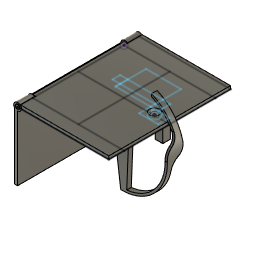
useless_machine (Autodesk Fusion 360 design; units mm, degrees)
Autodesk Fusion 360 part; units mm, degrees
sketch "Sketch1" plane through (0, 0, 0) normal (0, 0, 1) x (1, 0, 0)
  line L0 (0, 0) -> (60, 0)
  line L1 (60, 0) -> (60, -60)
  line L2 (60, -60) -> (0, -60)
  line L3 (0, -60) -> (0, 0)
  line L4 (60, -30) -> (0, -30)
  line L5 (30, 0) -> (30, -60)
  circle A0 centre (50, -30) radius 3.25
  line L6 (60, 0) -> (60, 10)
  line L7 (60, 10) -> (0, 10)
  line L8 (0, 10) -> (0, 0)
  line L9 (60, -60) -> (60, -70)
  line L10 (60, -70) -> (0, -70)
  line L11 (0, -70) -> (0, -60)
  line L12 (56.25, -26.25) -> (43.75, -26.25)
  line L13 (43.75, -26.25) -> (43.75, -33.75)
  line L14 (43.75, -33.75) -> (56.25, -33.75)
  line L15 (56.25, -33.75) -> (56.25, -26.25)
  line L16 (43.75, -26.25) -> (43.75, -23.25)
  line L17 (43.75, -23.25) -> (48.75, -23.25)
  line L18 (48.75, -23.25) -> (48.75, -18.25)
  line L19 (48.75, -18.25) -> (43.75, -18.25)
  line L20 (43.75, -18.25) -> (43.75, -23.25)
  line L21 (48.75, -23.25) -> (48.75, -26.25)
  line L22 (43.75, -23.25) -> (20.75, -23.25)
  line L23 (20.75, -23.25) -> (20.75, -18.25)
  line L24 (20.75, -18.25) -> (15.75, -18.25)
  line L25 (15.75, -18.25) -> (15.75, -23.25)
  line L26 (15.75, -23.25) -> (20.75, -23.25)
  line L27 (43.75, -26.25) -> (20.75, -26.25)
  line L28 (20.75, -26.25) -> (20.75, -23.25)
  line L29 (43.75, -18.25) -> (20.75, -18.25)
  line L30 (20.75, -26.25) -> (20.75, -6.25)
  line L31 (20.75, -6.25) -> (43.75, -6.25)
  line L32 (43.75, -6.25) -> (43.75, -18.25)
  dimension "d2" = 60
  dimension "d3" = 60
  dimension "d36" = 10
  dimension "d37" = 10
  dimension "d66" = 12.5
  dimension "d71" = 3
  dimension "d72" = 5
  dimension "d73" = 5
  dimension "d74" = 23
  dimension "d75" = 5
  dimension "d76" = 5
  dimension "d77" = 20
  dimension "d78" = 23
  constraint coincident L0.start L3.end
  constraint horizontal L0
  constraint perpendicular L0 L1
  constraint perpendicular L1 L2
  constraint midpoint L1 L4.start
  constraint midpoint L3 L4.end
  constraint midpoint L0 L5.start
  constraint midpoint L2 L5.end
  constraint coincident L4 A0.centre
  constraint perpendicular L0 L6
  constraint perpendicular L6 L7
  constraint perpendicular L0 L8
  constraint perpendicular L2 L9
  constraint perpendicular L9 L10
  constraint perpendicular L2 L11
  constraint perpendicular L12 L16
  constraint perpendicular L13 L17
  constraint perpendicular L12 L18
  constraint perpendicular L18 L19
  constraint perpendicular L17 L20
  constraint coincident L12 L21.end
  constraint perpendicular L12 L21
  constraint perpendicular L16 L22
  constraint perpendicular L22 L23
  constraint perpendicular L23 L24
  constraint perpendicular L22 L25
  constraint perpendicular L23 L26
  constraint perpendicular L23 L27
  constraint perpendicular L26 L28
  constraint perpendicular L23 L29
  constraint perpendicular L29 L30
  constraint perpendicular L20 L31
  measures "d2" distance of L0.end L1.end
  measures "d3" distance of L1.end L2.end
  measures "d36" distance of L0.end L6.end
  measures "d37" distance of L1.end L9.end
  measures "d66" distance of L12.start L12.end
  measures "d71" distance of L12.end L16.end
  measures "d72" distance of L16.end L17.end
  measures "d73" distance of L17.end L18.end
  measures "d74" distance of L16.end L22.end
  measures "d75" distance of L22.end L23.end
  measures "d76" distance of L23.end L24.end
  measures "d77" distance of L27.end L30.end
  measures "d78" distance of L30.end L31.end
sketch "Sketch2" plane through (0, 0, 0) normal (0, 1, 0) x (1, 0, 0)
  line L0 (0, 0) -> (60, 0)
  line L1 (53, -5) -> (47, -5)
  line L2 (47, -5) -> (47, 0)
  line L3 (53, -5) -> (53, 0)
  line L4 (48.5, -5) -> (46.0621, -15.7265)
  line L5 (46.0621, -15.7265) -> (48.9875, -16.3913)
  line L6 (48.9875, -16.3913) -> (51.5765, -5)
  line L7 (60, 0) -> (60, -2)
  line L8 (60, -2) -> (0, -2)
  line L9 (50, 0) -> (50, 15)
  line L10 (50, 15) -> (43.65, 15)
  line L11 (50, 15) -> (56.35, 15)
  line L12 (43.65, 15) -> (43.65, 0)
  line L13 (56.35, 15) -> (56.35, 0)
  line L14 (60, 0) -> (60, 5)
  line L15 (60, 5) -> (0, 5)
  line L16 (0, 5) -> (0, 0)
  line L17 (50, -11.9367) -> (50, 0)
  line L18 (50.0011, -14.9682) -> (50.0011, -12.9457)
  arc A0 (61.1474, 22.757) -> (27.4271, 34.949) centre (37.6519, 10.501) ccw
  line L19 (0, 0) -> (0, 60)
  line L20 (-2, 0) -> (-2, 60)
  line L21 (0, 60) -> (-2, 60)
  circle A1 centre (0, 0) radius 2.5
  circle A2 centre (0, 0) radius 1.5
  circle A3 centre (0, 0) radius 1.25
  line L22 (0, 5) -> (0, -5.5)
  line L23 (4, 0) -> (-6, 0)
  circle A4 centre (0, 0) radius 2.75
  line L24 (61.1474, 22.757) -> (70.1289, 5.5376)
  line L25 (50.0011, -12.9457) -> (67.1852, -3.8928)
  line L26 (50.0011, -14.9682) -> (74.2155, -2.3382)
  line L27 (62.7118, 23.5761) -> (72.1211, 5.5949)
  line L28 (74.2155, -2.3382) -> (68.742, -5.2024)
  arc A5 (67.1852, -3.8928) -> (70.1289, 5.5376) centre (63.9225, 2.3004) ccw
  arc A6 (68.742, -5.2024) -> (72.1211, 5.5949) centre (65.0329, 1.8858) ccw
  arc A7 (50.0011, -14.9682) -> (51.4624, -14.206) centre (37.663, 10.4685) ccw
  arc A8 (62.7118, 23.5761) -> (22.7658, 34.4962) centre (37.663, 10.4685) ccw
  line L29 (43.65, 0) -> (37.15, 0)
  circle A9 centre (37.6519, 10.501) radius 3.5
  circle A10 centre (37.663, 10.4685) radius 4.5
  circle A11 centre (29.5538, 26.0146) radius 2
  line L30 (31.2409, 27.0886) -> (40.6044, 12.3806)
  circle A12 centre (29.5538, 26.0146) radius 3
  line L31 (32.0852, 27.6245) -> (41.4601, 12.8834)
  line L32 (34.4218, 9.1533) -> (27.708, 25.2444)
  line L33 (33.5097, 8.7363) -> (26.785, 24.8597)
  line L34 (32.0852, 27.6245) -> (27.4271, 34.949)
  line L35 (26.785, 24.8597) -> (22.7658, 34.4962)
  dimension "d11" = 11
  dimension "d12" = 3
  dimension "d15" = 2
  dimension "d18" = 15
  dimension "d19" = 6.35
  dimension "d20" = 6.35
  dimension "d21" = 5
  dimension "d24" = 53
  dimension "d28" = 60
  dimension "d29" = 2
  dimension "d30" = 60
  dimension "d31" = 5
  dimension "d32" = 3
  dimension "d33" = 2.5
  dimension "d52" = 5.5
  dimension "d58" = 7
  dimension "d59" = 8
  dimension "d61" = 6.5
  dimension "d107" = 7
  dimension "d108" = 9
  dimension "d110" = 4
  dimension "d111" = 6
  constraint perpendicular L1 L2
  constraint coincident L0 L3.end
  constraint perpendicular L0 L3
  constraint coincident L1 L4.start
  constraint perpendicular L4 L5
  constraint coincident L1 L6.end
  constraint perpendicular L5 L6
  constraint coincident L0.end L7.start
  constraint perpendicular L0 L7
  constraint perpendicular L2 L8
  constraint coincident L0 L9.start
  constraint perpendicular L0 L9
  constraint perpendicular L9 L10
  constraint perpendicular L9 L11
  constraint perpendicular L8 L12
  constraint coincident L0 L12.end
  constraint coincident L0 L13.end
  constraint perpendicular L0 L13
  constraint perpendicular L0 L14
  constraint perpendicular L13 L15
  constraint coincident L0.start L16.end
  constraint perpendicular L0 L16
  constraint parallel L17 L18
  constraint coincident L6 L17.start
  constraint perpendicular L0 L19
  constraint perpendicular L15 L22
  constraint coincident L0 L23.start
  constraint parallel L0 L23
  constraint concentric A2 A4
  constraint coincident L27.start A7
  constraint tangent A0 L25
  constraint perpendicular L24 L26
  constraint tangent L27 A7
  constraint perpendicular L27 L28
  constraint tangent L25 A5
  constraint tangent L24 A5
  constraint tangent L28 A6
  constraint tangent L27 A6
  constraint concentric A7 A8
  constraint coincident L26 A7.end
  constraint concentric A8 A10
  constraint tangent A11 L30
  constraint coincident A9 L30.end
  constraint tangent A9 L30
  constraint coincident A11 L30.start
  constraint concentric A11 A12
  constraint tangent A10 L31
  constraint tangent A12 L31
  constraint coincident A12 L31.start
  constraint coincident A9 L32.start
  constraint tangent A10 L33
  constraint tangent A12 L33
  constraint coincident A12 L33.end
  constraint coincident A10 L33.start
  constraint parallel L31 L34
  constraint tangent A12 L35
  constraint coincident A10 L31.end
  measures "d11" distance of L4.start L4.end
  measures "d12" distance of L4.end L5.end
  measures "d15" distance of L0.end L7.end
  measures "d18" distance of L9.start L9.end
  measures "d19" distance of L9.end L10.end
  measures "d20" distance of L9.end L11.end
  measures "d21" distance of L0.end L14.end
  measures "d24" diameter of A0
  measures "d28" distance of L0.start L19.end
  measures "d29" distance of L0.start L20.start
  measures "d30" distance of L20.start L20.end
  measures "d31" diameter of A1
  measures "d32" diameter of A2
  measures "d33" diameter of A3
  measures "d52" diameter of A4
  measures "d58" radius of A5
  measures "d59" radius of A6
  measures "d61" distance of L12.end L29.end
  measures "d107" diameter of A9
  measures "d108" diameter of A10
  measures "d110" diameter of A11
  measures "d111" diameter of A12
extrude "돌출11" add sketch "Sketch1" against normal blind 8 contours L5 L29 L31 L32 | L5 L29 L30 L31 | L5 L20 L22 L29 | L5 L22 L23 L29 L30 makes body 1
extrude "돌출12" add sketch "Sketch2" against normal blind 70 contours L0 L2 L8 L23 A4 L29 | L0 L2 L8 L17 | L0 L3 L8 L17 | L0 L3 L7 L8 bodies 1
extrude "돌출13" add 1 faces at (40.9167, 0, 0.6667) along direction (0, 1, 0) blind 10 on bodies 1 bodies 1
extrude "돌출14" add sketch "Sketch1" against normal blind 20 contours L17 L18 L19 L20 | L23 L24 L25 L26 L30 bodies 1
extrude "돌출15" cut sketch "Sketch1" along normal blind 7 contours L4 A0 | L4 A0 bodies 1
extrude "돌출16" add sketch "Sketch2" against normal blind 60 contours L0 A3 L22 L23 | L0 A2 A3 L22 L23 | L0 L8 A1 A2 L22 L23 | L0 L8 A1 L23 A4 bodies 1
extrude "돌출17" add sketch "Sketch2" against normal blind 70 contours L0 L16 L19 A3 L22 L23 | L16 L19 A3 L22 L23 | L0 A3 L22 L23 | A3 L22 L23 bodies 1
extrude "돌출18" add sketch "Sketch2" along normal blind 10 contours L0 L16 L19 A3 L22 L23 | L16 L19 A3 L22 L23 | L0 A3 L22 L23 | A3 L22 L23 bodies 1
extrude "돌출19" add sketch "Sketch2" along normal blind 10 separate body contours L0 L16 L19 A1 A2 L22 L23 | L0 L8 A1 A2 L22 L23 | L16 L19 L20 A1 A2 L22 L23 | A1 A2 L22 L23 | L16 L19 L20 A1 L22 A4 | L8 A1 L22 | L20 A1 L23 | L16 L19 L20 L21 L22 A4 makes body 2
extrude "돌출20" add sketch "Sketch2" against normal blind 23.25 contours L0 L16 L19 A1 A2 L22 L23 | L0 L8 A1 A2 L22 L23 | L16 L19 L20 A1 A2 L22 L23 | A1 A2 L22 L23 | L16 L19 L20 A1 L22 A4 | L8 A1 L22 | L20 A1 L23 | L16 L19 L20 L21 L22 A4 bodies 2
extrude "돌출21" add 1 faces at (-1.3333, -23.25, -22.2958) along direction (0, -1, 0) blind 46.75 on bodies 2 bodies 2
extrude "돌출22" cut sketch "Sketch2" along normal blind 0.5 contours L0 L16 L19 A1 A2 L22 L23 | L0 L8 A1 A2 L22 L23 | A1 A2 L22 L23 | L8 A1 L22 bodies 2
extrude "돌출23" cut 1 faces at (2.1617, 0, -0.0408) along direction (0, -1, 0) blind 60.5 on bodies 2 bodies 2
extrude "돌출24" cut 1 faces at (-0.6667, -43.3333, -60) along direction (0, 0, 1) blind 15 on bodies 2 bodies 2
sketch "스케치3" plane through (0, -23.25, 0) normal (0, -1, 0) x (1, 0, 0)
  line L0 (48.75, 0) -> (15.75, 0)
  line L1 (15.75, 0) -> (15.75, -20)
  line L2 (15.75, -20) -> (20.75, -20)
  line L3 (20.75, -20) -> (20.75, -8)
  line L4 (20.75, -8) -> (43.75, -8)
  line L5 (43.75, -8) -> (43.75, -20)
  line L6 (43.75, -20) -> (48.75, -20)
  line L7 (48.75, -20) -> (48.75, 0)
  line L8 (34.2798, -14.4754) -> (36.5111, -31.7676)
  line L9 (33.2814, -14.5703) -> (35.5194, -31.896)
  line L10 (40.4928, -31.5983) -> (41.2478, -14.179)
  line L11 (41.4919, -31.6402) -> (42.2402, -14.1866)
  line L12 (41.4919, -31.6402) -> (41.1201, -40.3124)
  line L13 (35.5194, -31.896) -> (36.8569, -42.251)
  line L14 (41.1201, -40.3124) -> (41.0347, -42.3032)
  line L15 (36.8569, -42.251) -> (37.0811, -43.9865)
  line L16 (50, 13.3887) -> (50, 11.7365)
  arc A0 (37.0811, -43.9865) -> (50, 13.3887) centre (37.7444, -13.9938) ccw
  arc A1 (41.0347, -42.3032) -> (50, 11.7365) centre (37.7444, -13.9938) ccw
  line L17 (66.2183, -12.7742) -> (67.7169, -12.7101)
  arc A2 (40.4928, -31.5983) -> (36.5111, -31.7676) centre (38.4947, -31.5117) cw
  arc A3 (33.2814, -14.5703) -> (42.2402, -14.1866) centre (37.7444, -13.9938) cw
  arc A4 (34.2798, -14.4754) -> (41.2478, -14.179) centre (37.751, -14.0275) cw
  point P0 (37.7444, -13.9938)
  dimension "d114" = 7
  dimension "d115" = 9
  dimension "d116" = 4
  dimension "d118" = 57
  dimension "d119" = 60
  constraint tangent L10 A2
  constraint tangent L10 A4
  constraint tangent L11 A3
  constraint tangent L9 A3
  constraint parallel L11 L12
  constraint concentric A1 A3
  constraint concentric A0 A3
  constraint parallel L12 L14
  constraint parallel L13 L15
  constraint vertical L16
  constraint coincident A1 L17.start
  constraint coincident A0 L17.end
  measures "d114" diameter of A4
  measures "d115" diameter of A3
  measures "d116" diameter of A2
  measures "d118" diameter of A1
  measures "d119" diameter of A0
extrude "돌출25" add sketch "스케치3" against normal blind 3 separate body contours L9 L11 L12 L13 L14 L15 A0 A1 L17 A3 makes body 3
extrude "돌출26" add sketch "스케치3" against normal blind 1 contours L8 L10 A2 A4 bodies 3
move_body "이동1" bodies 3 to x (1, 0, 0) y (0, 1, 0) z (0, 0, 1) at (0, -16, 0)
extrude "돌출27" add sketch "스케치3" along normal blind 16 contours L16 A0 A1 L17 bodies 3
extrude "돌출28" cut sketch "스케치3" along normal blind 5 contours L16 A0 A1 L17 bodies 3
sketch "스케치4" plane through (0, -39.25, 0) normal (0, -1, 0) x (1, 0, 0)
  line L0 (33.2814, -14.5703) -> (37.0811, -43.9865)
  arc A0 (37.0811, -43.9865) -> (50, 13.3887) centre (37.7444, -13.9938) ccw
  line L1 (50, 13.3887) -> (50, 11.7365)
  arc A1 (41.0347, -42.3032) -> (50, 11.7365) centre (37.7444, -13.9938) ccw
  line L2 (41.0347, -42.3032) -> (42.2402, -14.1866)
  arc A2 (42.2402, -14.1866) -> (33.2814, -14.5703) centre (37.7444, -13.9938) ccw
  line L3 (67.7196, -12.7744) -> (67.1007, -7.8129)
  line L4 (67.1007, -7.8129) -> (65.6068, -7.9992)
  dimension "d128" = 5
  constraint coincident A0 L3.start
  constraint coincident A0 L3.end
  constraint coincident A1 L4.end
  constraint perpendicular L3 L4
  measures "d128" distance of L3.start L3.end
extrude "돌출29" cut sketch "스케치4" against normal blind 7.35 contours A0 L1 A1 L4 bodies 3
fillet "모깎기1" radius 7 4 edges at (66.9676, -28.25, -12.7421) (66.3538, -31.9, -7.906) (66.3538, -39.25, -7.906) (66.9676, -36.25, -12.7421) on bodies 3
extrude "Extrude1" [suppressed]
extrude "Extrude2" [suppressed]
extrude "Extrude3" [suppressed]
extrude "Extrude4" [suppressed]
extrude "Extrude5" [suppressed]
extrude "Extrude6" [suppressed]
extrude "Extrude7" [suppressed]
extrude "Extrude8" [suppressed]
extrude "Extrude9" [suppressed]
extrude "Extrude10" [suppressed]
